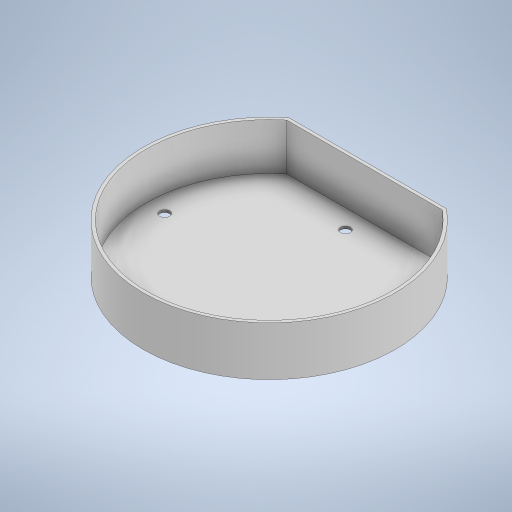
# Autodesk Inventor part: Casco
Saved by Autodesk Inventor 2024.2 (Build 282272000, 272)
## iProperties
Created: 2023-12-14
Part Number: Casco
Material: Generic
Document SubType Name: Modeling
Designer: felip
Density: 1 g/cm^3
Appearance: Default
Author: felip
Autodesk Inventor part; units mm, degrees
ref_plane "YZ Plane" through (0, 0, 0) normal (1, 0, 0) x (0, 1, 0)
ref_plane "XZ Plane" through (0, 0, 0) normal (0, 1, 0) x (-1, 0, 0)
ref_plane "XY Plane" through (0, 0, 0) normal (0, 0, 1) x (1, 0, 0)
sketch "Sketch1" plane through (0, 0, 0) normal (0, 1, 0) x (-1, 0, 0)
  circle A0 centre (0, 0) radius 102.5
  line L0 (0, 0) -> (85, 0)
  line L1 (0, 0) -> (0, -62)
  line L2 (0, 0) -> (-85, 0)
  line L3 (0, 0) -> (0, 85)
  circle A1 centre (-85, 0) radius 4
  circle A2 centre (0, -62) radius 4
  circle A3 centre (85, 0) radius 4
  circle A4 centre (0, 85) radius 4
  circle A5 centre (0, 0) radius 100
  dimension "d0" = 205
  dimension "d1" = 85
  dimension "d2" = 62
  dimension "d3" = 85
  dimension "d4" = 85
  dimension "d5" = 8
  dimension "d6" = 8
  dimension "d7" = 8
  dimension "d8" = 8
  dimension "d9" = 200
  constraints: 8 end point, 6 centre point, 6 coincident, 2 horizontal, 2 vertical
  measures "d0" diameter of A0
  measures "d1" distance of L0.start L0.end
  measures "d2" distance of L0.start L1.end
  measures "d3" distance of L0.start L2.end
  measures "d4" distance of L0.start L3.end
  measures "d5" diameter of A1
  measures "d6" diameter of A2
  measures "d7" diameter of A3
  measures "d8" diameter of A4
  measures "d9" diameter of A5
extrude "Extrusion1" add sketch "Sketch1" along normal blind 2 contours A5
extrude "Extrusion2" add sketch "Sketch1" along normal blind 40 contours A0
sketch "Sketch5" plane through (0, 0, 0) normal (0, -1, 0) x (1, 0, 0)
  line L0 (0, 0) -> (0, -80)
  line L1 (0, -80) -> (64.08, -80)
  circle A0 centre (0, 0) radius 102.5 projected
  line L2 (0, -80) -> (-64.08, -80)
  arc A1 (-64.08, -80) -> (64.08, -80) centre (0, 0) ccw
  dimension "d24" = 80
  constraints: 6 end point, 4 point on circle, 1 centre point, 1 concentric, 1 perpendicular, 1 point on line, 1 vertical
  measures "d24" distance of L0.start L0.end
extrude "Extrusion5" cut sketch "Sketch5" against normal blind 40 contours L1 A0 L2 picked at (38.9345, -82.6335)
sketch "Sketch7" plane through (64.08, 0, -80) normal (0, 0, -1) x (-1, 0, 0)
  line L0 (128.1601, 0) -> (0, 0)
  line L1 (0, 0) -> (0, 40)
  line L2 (0, 40) -> (128.1601, 40)
  line L3 (128.1601, 40) -> (128.1601, 0)
  line L4 (166.58, 0) -> (-38.42, 0) projected
  point P0 (64.08, 0)
  constraints: 8 end point, 2 parallel, 1 collinear, 1 perpendicular
extrude "Extrusion7" add sketch "Sketch7" against normal blind 2.5
sketch "Sketch8" plane through (64.08, 0, -80) normal (0, 0, -1) x (-1, 0, 0)
  line L0 (83.8335, 1.1684) -> (40.1844, 1.1684) construction
  line L1 (40.1844, 1.1684) -> (40.1844, 7.6688) construction
  line L2 (40.1844, 7.6688) -> (83.8335, 7.6688) construction
  line L3 (83.8335, 7.6688) -> (83.8335, 1.1684) construction
  line L4 (78.4948, 7.5403) -> (79.5477, 7.5403)
  line L5 (79.5477, 7.5403) -> (81.4756, 5.1132)
  line L6 (81.4756, 5.1132) -> (82.4049, 5.1132)
  line L7 (82.4049, 5.1132) -> (82.4049, 7.5403)
  line L8 (82.4049, 7.5403) -> (83.2156, 7.5403)
  line L9 (83.2156, 7.5403) -> (83.2156, 1.4403)
  line L10 (83.2156, 1.4403) -> (81.6436, 1.4403)
  spline S0 degree 2 poles (81.6436, 1.4403) (81.1197, 1.4403) (80.4128, 1.554) (80.0915, 1.7616) knots 0 0 0 1 2 2 2
  spline S1 degree 2 poles (80.0915, 1.7616) (79.7701, 1.9692) (79.3994, 2.6168) (79.3994, 3.0963) knots 0 0 0 1 2 2 2
  spline S2 degree 2 poles (79.3994, 3.0963) (79.3994, 3.7636) (80.0816, 4.6683) (80.6649, 4.8858) knots 0 0 0 1 2 2 2
  line L11 (80.6649, 4.8858) -> (78.4948, 7.5403)
  spline S3 degree 2 poles (80.2447, 3.1606) (80.2447, 2.8936) (80.4325, 2.4833) (80.6303, 2.3499) knots 0 0 0 1 2 2 2
  spline S4 degree 2 poles (80.6303, 2.3499) (80.8033, 2.2362) (81.263, 2.1423) (81.5992, 2.1423) knots 0 0 0 1 2 2 2
  line L12 (81.5992, 2.1423) -> (82.4049, 2.1423)
  line L13 (82.4049, 2.1423) -> (82.4049, 4.4359)
  line L14 (82.4049, 4.4359) -> (81.6931, 4.4359)
  spline S5 degree 2 poles (81.6931, 4.4359) (81.3421, 4.4359) (80.7835, 4.3123) (80.5907, 4.1196) knots 0 0 0 1 2 2 2
  spline S6 degree 2 poles (80.5907, 4.1196) (80.4128, 3.9515) (80.2447, 3.4769) (80.2447, 3.1606) knots 0 0 0 1 2 2 2
  spline S7 degree 2 poles (76.0825, 7.6441) (77.1799, 7.6441) (78.386, 6.4132) (78.386, 5.2763) knots 0 0 0 1 2 2 2
  spline S8 degree 2 poles (78.386, 5.2763) (78.386, 4.1591) (77.2145, 2.8343) (76.2703, 2.8343) knots 0 0 0 1 2 2 2
  spline S9 degree 2 poles (76.2703, 2.8343) (75.8452, 2.8343) (75.1877, 3.0815) (74.9455, 3.3435) knots 0 0 0 1 2 2 2
  spline S10 degree 2 poles (74.9455, 3.3435) (74.6983, 3.6055) (74.4364, 4.3618) (74.4364, 4.9105) knots 0 0 0 1 2 2 2
  line L15 (74.4364, 4.9105) -> (74.4364, 5.3307)
  line L16 (74.4364, 5.3307) -> (77.605, 5.3307)
  spline S11 degree 2 poles (77.605, 5.3307) (77.605, 6.1265) (76.8042, 6.9718) (76.0923, 6.9718) knots 0 0 0 1 2 2 2
  spline S12 degree 2 poles (76.0923, 6.9718) (75.8402, 6.9718) (75.3509, 6.8581) (75.1531, 6.7692) knots 0 0 0 1 2 2 2
  spline S13 degree 2 poles (75.1531, 6.7692) (74.9455, 6.6703) (74.6588, 6.4973) (74.5649, 6.4182) knots 0 0 0 1 2 2 2
  line L17 (74.5649, 6.4182) -> (74.5204, 6.4182)
  line L18 (74.5204, 6.4182) -> (74.5204, 7.2585)
  spline S14 degree 2 poles (74.5204, 7.2585) (74.6539, 7.3129) (75.0592, 7.4711) (75.2174, 7.5156) knots 0 0 0 1 2 2 2
  spline S15 degree 2 poles (75.2174, 7.5156) (75.4398, 7.5799) (75.8056, 7.6441) (76.0825, 7.6441) knots 0 0 0 1 2 2 2
  spline S16 degree 2 poles (75.1877, 4.7424) (75.1976, 4.431) (75.3261, 3.9762) (75.4497, 3.823) knots 0 0 0 1 2 2 2
  spline S17 degree 2 poles (75.4497, 3.823) (75.5832, 3.65) (76.0034, 3.467) (76.3148, 3.467) knots 0 0 0 1 2 2 2
  spline S18 degree 2 poles (76.3148, 3.467) (76.6213, 3.467) (77.0513, 3.65) (77.2293, 3.8279) knots 0 0 0 1 2 2 2
  spline S19 degree 2 poles (77.2293, 3.8279) (77.4023, 4.0108) (77.5803, 4.4508) (77.605, 4.7424) knots 0 0 0 1 2 2 2
  line L19 (77.605, 4.7424) -> (75.1877, 4.7424)
  spline S20 degree 2 poles (71.1046, 7.0559) (71.1985, 7.1251) (71.5149, 7.3722) (71.6632, 7.4464) knots 0 0 0 1 2 2 2
  spline S21 degree 2 poles (71.6632, 7.4464) (71.8659, 7.5551) (72.2465, 7.6688) (72.5925, 7.6688) knots 0 0 0 1 2 2 2
  spline S22 degree 2 poles (72.5925, 7.6688) (72.8743, 7.6688) (73.3834, 7.4563) (73.5762, 7.2635) knots 0 0 0 1 2 2 2
  spline S23 degree 2 poles (73.5762, 7.2635) (73.7591, 7.0756) (73.9816, 6.522) (73.9816, 6.2155) knots 0 0 0 1 2 2 2
  spline S24 degree 2 poles (73.9816, 6.2155) (73.9816, 5.741) (73.5812, 5.0687) (73.1462, 4.8759) knots 0 0 0 1 2 2 2
  spline S25 degree 2 poles (73.1462, 4.8759) (72.7606, 4.6979) (71.7126, 4.5645) (71.1046, 4.5299) knots 0 0 0 1 2 2 2
  line L20 (71.1046, 4.5299) -> (71.1046, 4.3816)
  spline S26 degree 2 poles (71.1046, 4.3816) (71.1046, 4.1146) (71.2677, 3.7834) (71.416, 3.6895) knots 0 0 0 1 2 2 2
  spline S27 degree 2 poles (71.416, 3.6895) (71.5643, 3.5956) (71.9894, 3.5363) (72.2168, 3.5363) knots 0 0 0 1 2 2 2
  spline S28 degree 2 poles (72.2168, 3.5363) (72.4838, 3.5363) (73.2055, 3.6944) (73.5663, 3.8477) knots 0 0 0 1 2 2 2
  line L21 (73.5663, 3.8477) -> (73.6108, 3.8477)
  line L22 (73.6108, 3.8477) -> (73.6108, 3.0617)
  spline S29 degree 2 poles (73.6108, 3.0617) (73.3983, 3.0024) (72.6024, 2.8541) (72.2119, 2.8541) knots 0 0 0 1 2 2 2
  spline S30 degree 2 poles (72.2119, 2.8541) (71.7373, 2.8541) (71.0898, 3.0024) (70.8327, 3.1952) knots 0 0 0 1 2 2 2
  spline S31 degree 2 poles (70.8327, 3.1952) (70.5806, 3.383) (70.3334, 3.9812) (70.3334, 4.4112) knots 0 0 0 1 2 2 2
  line L23 (70.3334, 4.4112) -> (70.3334, 7.5403)
  line L24 (70.3334, 7.5403) -> (71.1046, 7.5403)
  line L25 (71.1046, 7.5403) -> (71.1046, 7.0559)
  line L26 (71.1046, 6.4132) -> (71.1046, 5.1428)
  spline S32 degree 2 poles (71.1046, 5.1428) (71.3814, 5.1675) (72.2168, 5.2516) (72.4788, 5.3307) knots 0 0 0 1 2 2 2
  spline S33 degree 2 poles (72.4788, 5.3307) (72.7853, 5.4246) (73.1857, 5.8151) (73.1857, 6.1611) knots 0 0 0 1 2 2 2
  spline S34 degree 2 poles (73.1857, 6.1611) (73.1857, 6.5566) (72.7408, 6.957) (72.3157, 6.957) knots 0 0 0 1 2 2 2
  spline S35 degree 2 poles (72.3157, 6.957) (71.9548, 6.957) (71.3616, 6.6456) (71.1046, 6.4132) knots 0 0 0 1 2 2 2
  line L27 (68.4649, 7.5403) -> (69.236, 7.5403)
  line L28 (69.236, 7.5403) -> (69.236, 1.1684)
  line L29 (69.236, 1.1684) -> (68.4649, 1.1684)
  line L30 (68.4649, 1.1684) -> (68.4649, 7.5403)
  line L31 (59.4236, 7.5403) -> (60.2343, 7.5403)
  line L32 (60.2343, 7.5403) -> (60.2343, 2.2856)
  line L33 (60.2343, 2.2856) -> (61.8261, 5.8596)
  line L34 (61.8261, 5.8596) -> (62.3204, 5.8596)
  line L35 (62.3204, 5.8596) -> (63.8973, 2.2856)
  line L36 (63.8973, 2.2856) -> (63.8973, 7.5403)
  line L37 (63.8973, 7.5403) -> (64.6536, 7.5403)
  line L38 (64.6536, 7.5403) -> (64.6536, 1.4403)
  line L39 (64.6536, 1.4403) -> (63.5463, 1.4403)
  line L40 (63.5463, 1.4403) -> (62.0238, 4.8363)
  line L41 (62.0238, 4.8363) -> (60.5507, 1.4403)
  line L42 (60.5507, 1.4403) -> (59.4236, 1.4403)
  line L43 (59.4236, 1.4403) -> (59.4236, 7.5403)
  spline S36 degree 2 poles (55.6964, 7.0559) (55.7903, 7.1251) (56.1067, 7.3722) (56.255, 7.4464) knots 0 0 0 1 2 2 2
  spline S37 degree 2 poles (56.255, 7.4464) (56.4577, 7.5551) (56.8383, 7.6688) (57.1843, 7.6688) knots 0 0 0 1 2 2 2
  spline S38 degree 2 poles (57.1843, 7.6688) (57.4661, 7.6688) (57.9753, 7.4563) (58.168, 7.2635) knots 0 0 0 1 2 2 2
  spline S39 degree 2 poles (58.168, 7.2635) (58.3509, 7.0756) (58.5734, 6.522) (58.5734, 6.2155) knots 0 0 0 1 2 2 2
  spline S40 degree 2 poles (58.5734, 6.2155) (58.5734, 5.741) (58.173, 5.0687) (57.738, 4.8759) knots 0 0 0 1 2 2 2
  spline S41 degree 2 poles (57.738, 4.8759) (57.3524, 4.6979) (56.3044, 4.5645) (55.6964, 4.5299) knots 0 0 0 1 2 2 2
  line L44 (55.6964, 4.5299) -> (55.6964, 4.3816)
  spline S42 degree 2 poles (55.6964, 4.3816) (55.6964, 4.1146) (55.8595, 3.7834) (56.0078, 3.6895) knots 0 0 0 1 2 2 2
  spline S43 degree 2 poles (56.0078, 3.6895) (56.1561, 3.5956) (56.5812, 3.5363) (56.8086, 3.5363) knots 0 0 0 1 2 2 2
  spline S44 degree 2 poles (56.8086, 3.5363) (57.0756, 3.5363) (57.7973, 3.6944) (58.1582, 3.8477) knots 0 0 0 1 2 2 2
  line L45 (58.1582, 3.8477) -> (58.2026, 3.8477)
  line L46 (58.2026, 3.8477) -> (58.2026, 3.0617)
  spline S45 degree 2 poles (58.2026, 3.0617) (57.9901, 3.0024) (57.1942, 2.8541) (56.8037, 2.8541) knots 0 0 0 1 2 2 2
  spline S46 degree 2 poles (56.8037, 2.8541) (56.3291, 2.8541) (55.6816, 3.0024) (55.4245, 3.1952) knots 0 0 0 1 2 2 2
  spline S47 degree 2 poles (55.4245, 3.1952) (55.1724, 3.383) (54.9253, 3.9812) (54.9253, 4.4112) knots 0 0 0 1 2 2 2
  line L47 (54.9253, 4.4112) -> (54.9253, 7.5403)
  line L48 (54.9253, 7.5403) -> (55.6964, 7.5403)
  line L49 (55.6964, 7.5403) -> (55.6964, 7.0559)
  line L50 (55.6964, 6.4132) -> (55.6964, 5.1428)
  spline S48 degree 2 poles (55.6964, 5.1428) (55.9732, 5.1675) (56.8086, 5.2516) (57.0706, 5.3307) knots 0 0 0 1 2 2 2
  spline S49 degree 2 poles (57.0706, 5.3307) (57.3771, 5.4246) (57.7775, 5.8151) (57.7775, 6.1611) knots 0 0 0 1 2 2 2
  spline S50 degree 2 poles (57.7775, 6.1611) (57.7775, 6.5566) (57.3326, 6.957) (56.9075, 6.957) knots 0 0 0 1 2 2 2
  spline S51 degree 2 poles (56.9075, 6.957) (56.5466, 6.957) (55.9535, 6.6456) (55.6964, 6.4132) knots 0 0 0 1 2 2 2
  line L51 (50.3231, 7.5403) -> (51.0942, 7.5403)
  line L52 (51.0942, 7.5403) -> (51.0942, 7.0756)
  spline S52 degree 2 poles (51.0942, 7.0756) (51.2722, 7.2239) (51.5342, 7.4217) (51.7121, 7.5057) knots 0 0 0 1 2 2 2
  spline S53 degree 2 poles (51.7121, 7.5057) (51.8753, 7.5848) (52.2262, 7.6688) (52.4586, 7.6688) knots 0 0 0 1 2 2 2
  spline S54 degree 2 poles (52.4586, 7.6688) (52.8342, 7.6688) (53.467, 7.3574) (53.6894, 7.0559) knots 0 0 0 1 2 2 2
  spline S55 degree 2 poles (53.6894, 7.0559) (53.9119, 6.7543) (54.159, 5.8645) (54.159, 5.2862) knots 0 0 0 1 2 2 2
  spline S56 degree 2 poles (54.159, 5.2862) (54.159, 4.6831) (53.8476, 3.8032) (53.5757, 3.472) knots 0 0 0 1 2 2 2
  spline S57 degree 2 poles (53.5757, 3.472) (53.3236, 3.1754) (52.6167, 2.8343) (52.2262, 2.8343) knots 0 0 0 1 2 2 2
  spline S58 degree 2 poles (52.2262, 2.8343) (51.8851, 2.8343) (51.376, 2.9876) (51.0942, 3.1457) knots 0 0 0 1 2 2 2
  line L53 (51.0942, 3.1457) -> (51.0942, 1.1684)
  line L54 (51.0942, 1.1684) -> (50.3231, 1.1684)
  line L55 (50.3231, 1.1684) -> (50.3231, 7.5403)
  line L56 (51.0942, 6.4281) -> (51.0942, 3.7834)
  spline S59 degree 2 poles (51.0942, 3.7834) (51.3809, 3.645) (51.8357, 3.5412) (52.0977, 3.5412) knots 0 0 0 1 2 2 2
  spline S60 degree 2 poles (52.0977, 3.5412) (52.6909, 3.5412) (53.3632, 4.431) (53.3632, 5.2713) knots 0 0 0 1 2 2 2
  spline S61 degree 2 poles (53.3632, 5.2713) (53.3632, 6.082) (52.8491, 6.9372) (52.2806, 6.9372) knots 0 0 0 1 2 2 2
  spline S62 degree 2 poles (52.2806, 6.9372) (51.9791, 6.9372) (51.3661, 6.6604) (51.0942, 6.4281) knots 0 0 0 1 2 2 2
  line L57 (46.7787, 3.7884) -> (46.8183, 3.7884)
  spline S63 degree 2 poles (46.8183, 3.7884) (46.9073, 3.7636) (47.1, 3.7538) (47.2335, 3.7538) knots 0 0 0 1 2 2 2
  spline S64 degree 2 poles (47.2335, 3.7538) (47.5449, 3.7538) (48.1579, 4.0256) (48.4347, 4.2926) knots 0 0 0 1 2 2 2
  line L58 (48.4347, 4.2926) -> (48.4347, 7.5403)
  line L59 (48.4347, 7.5403) -> (49.2059, 7.5403)
  line L60 (49.2059, 7.5403) -> (49.2059, 2.9628)
  line L61 (49.2059, 2.9628) -> (48.4347, 2.9628)
  line L62 (48.4347, 2.9628) -> (48.4347, 3.645)
  spline S65 degree 2 poles (48.4347, 3.645) (48.0146, 3.2693) (47.3868, 2.9628) (47.0902, 2.9628) knots 0 0 0 1 2 2 2
  spline S66 degree 2 poles (47.0902, 2.9628) (46.9715, 2.9628) (46.8529, 2.9727) (46.7787, 2.9876) knots 0 0 0 1 2 2 2
  line L63 (46.7787, 2.9876) -> (46.7787, 3.7884)
  line L64 (45.3946, 7.5403) -> (46.1658, 7.5403)
  line L65 (46.1658, 7.5403) -> (46.1658, 2.9628)
  line L66 (46.1658, 2.9628) -> (45.3946, 2.9628)
  line L67 (45.3946, 2.9628) -> (45.3946, 7.5403)
  line L68 (45.3402, 2.2016) -> (46.2152, 2.2016)
  line L69 (46.2152, 2.2016) -> (46.2152, 1.4008)
  line L70 (46.2152, 1.4008) -> (45.3402, 1.4008)
  line L71 (45.3402, 1.4008) -> (45.3402, 2.2016)
  line L72 (40.743, 7.5403) -> (41.5141, 7.5403)
  line L73 (41.5141, 7.5403) -> (41.5141, 7.0756)
  spline S67 degree 2 poles (41.5141, 7.0756) (41.6921, 7.2239) (41.9541, 7.4217) (42.1321, 7.5057) knots 0 0 0 1 2 2 2
  spline S68 degree 2 poles (42.1321, 7.5057) (42.2952, 7.5848) (42.6462, 7.6688) (42.8785, 7.6688) knots 0 0 0 1 2 2 2
  spline S69 degree 2 poles (42.8785, 7.6688) (43.2542, 7.6688) (43.8869, 7.3574) (44.1094, 7.0559) knots 0 0 0 1 2 2 2
  spline S70 degree 2 poles (44.1094, 7.0559) (44.3318, 6.7543) (44.579, 5.8645) (44.579, 5.2862) knots 0 0 0 1 2 2 2
  spline S71 degree 2 poles (44.579, 5.2862) (44.579, 4.6831) (44.2676, 3.8032) (43.9957, 3.472) knots 0 0 0 1 2 2 2
  spline S72 degree 2 poles (43.9957, 3.472) (43.7436, 3.1754) (43.0367, 2.8343) (42.6462, 2.8343) knots 0 0 0 1 2 2 2
  spline S73 degree 2 poles (42.6462, 2.8343) (42.3051, 2.8343) (41.7959, 2.9876) (41.5141, 3.1457) knots 0 0 0 1 2 2 2
  line L74 (41.5141, 3.1457) -> (41.5141, 1.1684)
  line L75 (41.5141, 1.1684) -> (40.743, 1.1684)
  line L76 (40.743, 1.1684) -> (40.743, 7.5403)
  line L77 (41.5141, 6.4281) -> (41.5141, 3.7834)
  spline S74 degree 2 poles (41.5141, 3.7834) (41.8009, 3.645) (42.2556, 3.5412) (42.5176, 3.5412) knots 0 0 0 1 2 2 2
  spline S75 degree 2 poles (42.5176, 3.5412) (43.1108, 3.5412) (43.7831, 4.431) (43.7831, 5.2713) knots 0 0 0 1 2 2 2
  spline S76 degree 2 poles (43.7831, 5.2713) (43.7831, 6.082) (43.269, 6.9372) (42.7005, 6.9372) knots 0 0 0 1 2 2 2
  spline S77 degree 2 poles (42.7005, 6.9372) (42.399, 6.9372) (41.786, 6.6604) (41.5141, 6.4281) knots 0 0 0 1 2 2 2
  point P0 (64.08, 0)
  constraints: 2 other
extrude "Extrusion8" add sketch "Sketch8" along normal blind 1
body "Solid1"
